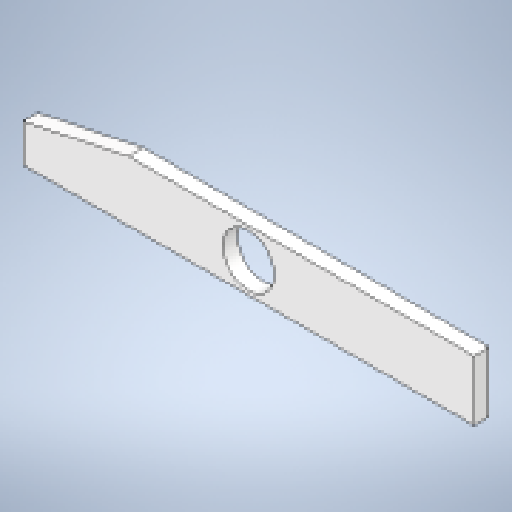
# Autodesk Inventor part: Side_Plate
Saved by Autodesk Inventor 2023.2 (Build 272271000, 271)
## iProperties
Created: 2024-01-26
Part Number: Side_Plate
Material: UHMW, White
Document SubType Name: Modeling
Designer: Nathan Cai
Density: 0.94 g/cm^3
Appearance: Smooth - White
Mass: 16.023 g
Surface Area: 76.6247 cm^2
Volume: 17.0458 cm^3
Author: Nathan Cai
Autodesk Inventor part; units mm, degrees
ref_plane "YZ Plane" through (0, 0, 0) normal (1, 0, 0) x (0, 1, 0)
ref_plane "XZ Plane" through (0, 0, 0) normal (0, 1, 0) x (-1, 0, 0)
ref_plane "XY Plane" through (0, 0, 0) normal (0, 0, 1) x (1, 0, 0)
sketch "Sketch1" plane through (0, 0, 0) normal (0, 0, 1) x (1, 0, 0)
  line L0 (0, 0) -> (120.65, 0)
  line L1 (120.65, 0) -> (120.65, 25.4)
  line L2 (120.65, 25.4) -> (0, 25.4)
  line L3 (0, 25.4) -> (0, 0)
  line L4 (0, 12.7) -> (120.65, 12.7) construction
  circle A0 centre (25.4, 12.7) radius 11
  point P0 (44.45, 25.4)
  dimension "d0" = 120.65
  dimension "d1" = 25.4
  dimension "d5" = 44.45
  dimension "d6" = 22
  dimension "d7" = 95.25
  constraints: 10 end point, 2 midpoint, 2 parallel, 2 point on line, 1 centre point, 1 horizontal, 1 perpendicular
  measures "d0" distance of L2.end L1.end
  measures "d1" distance of L1.end L0.end
  measures "d5" distance from line of L3 point (44.45, 25.4)
  measures "d6" diameter of A0
  measures "d7" distance from line of L1 A0.centre
extrude "Extrusion1" add sketch "Sketch1" along normal blind 6.35
body "Solid1"
